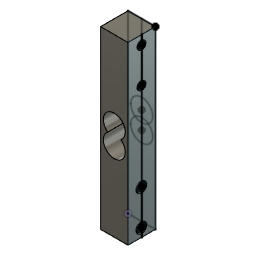
mixmeasurebuddy_v33 (Autodesk Fusion 360 archive; units mm, degrees)
design "wiegezelle"
Autodesk Fusion 360 part; units mm, degrees
sketch "Skizze1" plane through (0, 0, 0) normal (0, 1, 0) x (1, 0, 0)
  line L0 (0, 0) -> (12.5, 0)
  line L1 (12.5, 0) -> (12.5, -12.5)
  line L2 (12.5, -12.5) -> (0, -12.5)
  line L3 (0, -12.5) -> (0, 0)
  dimension "d1" = 12.5
  dimension "d2" = 12.5
  constraint horizontal L0
  constraint vertical L1
  constraint horizontal L2
  constraint vertical L3
  constraint coincident L0.start L3.end
  measures "d1" distance of L0.start L0.end
  measures "d2" distance of L0.start L2.end
extrude "Extrusion1" add sketch "Skizze1" along normal blind 80
sketch "Skizze2" plane through (12.5, 0, 0) normal (1, 0, 0) x (0, 0, -1)
  line L0 (-12.5, 0) -> (0, 0)
  line L1 (0, 0) -> (0, 80)
  line L2 (0, 80) -> (-12.5, 80)
  line L3 (-12.5, 80) -> (-12.5, 0)
  line L4 (-6.25, 80) -> (-6.25, 0)
  line L5 (-6.25, 80) -> (-6.25, 76)
  line L6 (-6.25, 80) -> (-6.25, 60)
  line L7 (-6.25, 0) -> (-6.25, 4)
  line L8 (-6.25, 0) -> (-6.25, 20)
  circle A0 centre (-6.25, 20) radius 1.65
  circle A1 centre (-6.25, 4) radius 1.65
  circle A2 centre (-6.25, 60) radius 1.65
  circle A3 centre (-6.25, 76) radius 1.65
  dimension "d5" = 4
  dimension "d6" = 20
  dimension "d7" = 4
  dimension "d8" = 20
  dimension "d9" = 3.3
  dimension "d10" = 3.3
  dimension "d11" = 3.3
  dimension "d12" = 3.3
  constraint midpoint L2 L4.start
  constraint midpoint L0 L4.end
  constraint perpendicular L0 L5
  constraint perpendicular L2 L6
  constraint vertical L7
  constraint perpendicular L0 L8
  constraint coincident L8.end A0.centre
  constraint coincident L7.end A1.centre
  constraint coincident L6.end A2.centre
  constraint coincident L5.end A3.centre
  measures "d5" distance of L4.start L5.end
  measures "d6" distance of L4.start L6.end
  measures "d7" distance of L4.end L7.end
  measures "d8" distance of L4.end L8.end
  measures "d9" diameter of A0
  measures "d10" diameter of A1
  measures "d11" diameter of A2
  measures "d12" diameter of A3
extrude "Extrusion2" cut sketch "Skizze2" against normal blind 19 contours L4 L7 L8 A1 | L4 L7 L8 A1 | L4 L5 L6 A3 | L4 L5 L6 A3 | L4 L8 A0 | L4 L8 A0 | L4 L6 A2 | L4 L6 A2
thread "Gewinde1" "ISO Metric profile 4.0 M4x0.7 6H" major diameter 4.1095 minor diameter 3.332 pitch 0.7 angle 60 modelled right hand crest width 0.193 on face at (8.3333, 76.6409, 7.7704) crest through (12.325, 76, 4.584)
thread "Gewinde2" "ISO Metric profile 4.0 M4x0.7 6H" major diameter 4.1095 minor diameter 3.332 pitch 0.7 angle 60 modelled right hand crest width 0.193 on face at (8.3333, 59.6731, 7.8673) crest through (12.325, 60, 4.584)
thread "Gewinde3" "ISO Metric profile 5.0 M5x0.8 6H" major diameter 5.12 minor diameter 4.234 pitch 0.8 angle 60 modelled right hand crest width 0.2219 on face at (4.1667, 19.9178, 4.6021) crest through (12.3, 20, 4.133)
thread "Gewinde4" "ISO Metric profile 5.0 M5x0.8 6H" major diameter 5.12 minor diameter 4.234 pitch 0.8 angle 60 modelled right hand crest width 0.2219 on face at (8.3333, 4.1643, 4.6082) crest through (12.3, 4, 4.133)
sketch "Skizze3" plane through (0, 0, 0) normal (0, 0, -1) x (-1, 0, 0)
  line L0 (-12.5, 0) -> (0, 0)
  line L1 (0, 0) -> (0, 80)
  line L2 (0, 80) -> (-12.5, 80)
  line L3 (-12.5, 80) -> (-12.5, 0)
  line L4 (-12.5, 80) -> (0, 80)
  line L5 (0, 80) -> (0, 0)
  line L6 (0, 0) -> (-12.5, 0)
  line L7 (-12.5, 0) -> (-12.5, 80)
  line L8 (-6.25, 80) -> (-6.25, 0)
  line L9 (-6.25, 40) -> (-6.25, 44)
  line L10 (-6.25, 40) -> (-6.25, 36)
  circle A0 centre (-6.25, 36) radius 5
  circle A1 centre (-6.25, 44) radius 5
  dimension "d15" = 4
  dimension "d16" = 4
  dimension "d17" = 10
  dimension "d18" = 10
  constraint horizontal L4
  constraint vertical L5
  constraint horizontal L6
  constraint vertical L7
  constraint coincident L0.end L1.start
  constraint coincident L2.end L3.start
  constraint midpoint L4 L8.start
  constraint midpoint L6 L8.end
  constraint midpoint L8 L9.start
  constraint parallel L8 L9
  constraint parallel L8 L10
  constraint coincident L10.end A0.centre
  constraint coincident L9.end A1.centre
  measures "d15" distance of L9.start L9.end
  measures "d16" distance of L9.start L10.end
  measures "d17" diameter of A0
  measures "d18" diameter of A1
extrude "Extrusion3" cut sketch "Skizze3" against normal blind 12.5 contours L8 L10 A0 A1 | L8 L10 A0 A1 | L8 L9 A0 A1 | L8 L9 L10 A0 A1 | L8 L9 A0 A1 | L8 L9 L10 A0 A1
